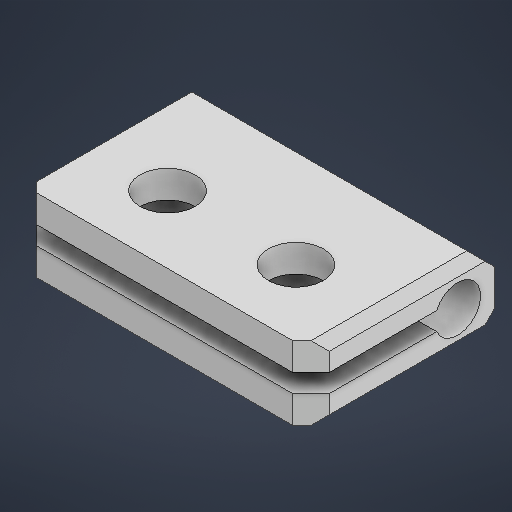
# Autodesk Inventor part: Sup_haste_corpo
Saved by Autodesk Inventor 2026.1 (Build 301233020, 233B)
## iProperties
Created: 2026-03-23
Part Number: Sup_haste_corpo
Material: Genérico
Document SubType Name: Modeling
Designer: celio
Density: 1 g/cm^3
Appearance: Padrão
Author: celio
Autodesk Inventor part; units mm, degrees
ref_plane "YZ Plane" through (0, 0, 0) normal (1, 0, 0) x (0, 1, 0)
ref_plane "XZ Plane" through (0, 0, 0) normal (0, 1, 0) x (-1, 0, 0)
ref_plane "XY Plane" through (0, 0, 0) normal (0, 0, 1) x (1, 0, 0)
sketch "Esboço1" plane through (0, 0, 0) normal (0, 1, 0) x (-1, 0, 0)
  line L0 (-8, -5) -> (8, -5)
  line L1 (8, -5) -> (8, 5)
  line L2 (8, 5) -> (-8, 5)
  line L3 (-8, 5) -> (-8, -5)
  line L4 (-8, -5) -> (8, 5) construction
  line L5 (8, -5) -> (-8, 5) construction
  point P0 (0, 0)
  dimension "d0" = 16
  dimension "d1" = 10
  constraints: 12 end point, 2 midpoint, 2 parallel, 1 horizontal, 1 perpendicular
  measures "d0" distance of L2.end L1.end
  measures "d1" distance of L1.end L0.end
extrude "Extrusão1" add sketch "Esboço1" along normal blind 4
sketch "Esboço2" plane through (8, 0, 5) normal (1, 0, 0) x (0, 0, -1)
  line L0 (0, 0) -> (0, 4) projected
  line L1 (10, 0) -> (10, 4) projected
  arc A0 (6.8544, 1.5) -> (6.8544, 2.5) centre (8, 2) ccw
  line L2 (-0.795, 1.5) -> (-0.795, 2.5)
  line L3 (-0.795, 2.5) -> (6.8544, 2.5)
  line L4 (6.8544, 1.5) -> (-0.795, 1.5)
  point P0 (5, 0)
  point P1 (0, 2.5)
  point P2 (0, 1.5)
  dimension "d7" = 2.5
  dimension "d8" = 1
  constraints: 6 end point, 2 point on circle, 1 centre point, 1 horizontal, 1 parallel, 1 perpendicular
  measures "d7" diameter of A0
  measures "d8" distance of L2.start L2.end
extrude "Extrusão2" cut sketch "Esboço2" against normal through all contours L0 L3 A0 L4
chamfer "Chanfro1" distance 1 angle 45 4 edges at (-8, 3.25, 5) (-8, 0.75, 5) (8, 0.75, 5) (8, 3.25, 5)
chamfer "Chanfro2" distance 1 angle 45 2 edges at (0, 4, -5) (0, 0, -5)
chamfer "Chanfro3" distance 0.5 angle 45 4 edges at (8, 4, 0) (8, 0, 0) (-8, 4, 0) (-8, 0, 0)
sketch "Esboço3" plane through (0, 4, 0) normal (0, 1, 0) x (1, 0, 0)
  line L0 (-7.5, -4.5) -> (-7.5, 4) projected
  line L1 (7, -5) -> (8, -4) projected
  line L2 (-7.5, 4) -> (7.5, 4)
  line L3 (7.5, 4) -> (7.5, -4.5)
  line L4 (7.5, -4.5) -> (-7.5, -4.5)
  line L5 (-7.5, -4.5) -> (-7.5, 4)
  line L6 (8, 1.8544) -> (-8, 1.8544) projected
  line L7 (-7.5, 1.8544) -> (7.5, 1.8544)
  line L8 (7.5, 1.8544) -> (7.5, -4.5)
  line L9 (7.5, -4.5) -> (-7.5, -4.5)
  line L10 (-7.5, -4.5) -> (-7.5, 1.8544)
  line L11 (-7.5, -1.3228) -> (7.5, -1.3228)
  line L12 (-7.5, -1.3228) -> (-3.5, -1.3228)
  circle A0 centre (-3.5, -1.3228) radius 1.5
  line L13 (7.5, -1.3228) -> (3.5, -1.3228)
  circle A1 centre (3.5, -1.3228) radius 1.5
  point P0 (0, 0)
  dimension "d20" = 4
  dimension "d21" = 3
  dimension "d22" = 4
  dimension "d23" = 3
  constraints: 22 end point, 4 parallel, 4 point on line, 3 midpoint, 2 centre point, 2 coincident, 2 horizontal, 2 perpendicular
  measures "d20" distance of L11.start L12.end
  measures "d21" diameter of A0
  measures "d22" distance of L11.end L13.end
  measures "d23" diameter of A1
extrude "Extrusão3" cut sketch "Esboço3" against normal through all contours A0 L11 | L11 A0 | A1 L11 | L11 A1
